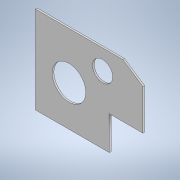
# Autodesk Inventor part: Assignment 1.2 - Spacer Plate
Saved by Autodesk Inventor 2021.1 (Build 251245000, 245)
## iProperties
Created: 2021-05-12
Part Number: Assignment 1.2 - Spacer Plate
Material: Generic
Document SubType Name: Modeling
Designer: as000166
Density: 1 g/cm^3
Appearance: Default
Author: as000166
Autodesk Inventor part; units mm, degrees
ref_plane "YZ Plane" through (0, 0, 0) normal (1, 0, 0) x (0, 1, 0)
ref_plane "XZ Plane" through (0, 0, 0) normal (0, 1, 0) x (-1, 0, 0)
ref_plane "XY Plane" through (0, 0, 0) normal (0, 0, 1) x (1, 0, 0)
sketch "Sketch1" plane through (0, 0, 0) normal (0, 0, 1) x (1, 0, 0)
  line L0 (0, 165.1) -> (165.1, 165.1)
  line L1 (165.1, 165.1) -> (203.2, 139.7)
  circle A0 centre (63.5, 76.2) radius 31.75
  line L2 (139.7, 0) -> (139.7, 63.5)
  line L3 (139.7, 63.5) -> (203.2, 63.5)
  line L4 (0, 0) -> (139.7, 0)
  line L5 (203.2, 63.5) -> (203.2, 139.7)
  circle A1 centre (127, 127) radius 19.05
  line L6 (0, 165.1) -> (0, 0)
  dimension "d2" = 165.1
  dimension "d3" = 165.1
  dimension "d6" = 63.5
  dimension "d8" = 63.5
  dimension "d11" = 38.1
  constraints: 14 end point, 2 centre point, 1 horizontal, 1 perpendicular, 1 vertical
  measures "d2" distance of L4.start L0.start
  measures "d3" distance of L0.start L0.end
  measures "d6" diameter of A0
  measures "d8" distance of L2.start L2.end
  measures "d11" diameter of A1
extrude "Extrusion1" add sketch "Sketch1" along normal blind 3.175
body "Solid1"
